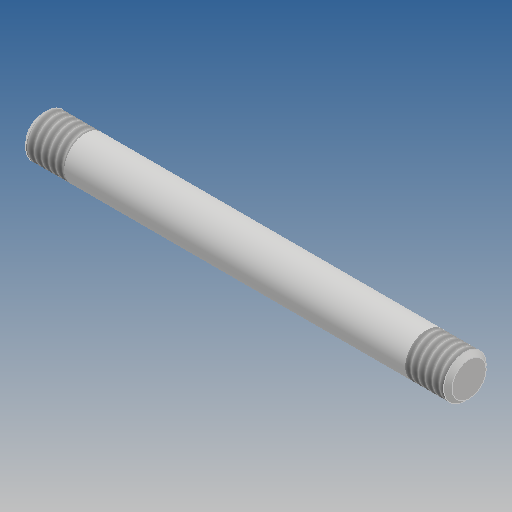
# Autodesk Inventor part: Pleuel
Saved by Autodesk Inventor 2018 (Build 220112000, 112)
## iProperties
Created: 2018-10-09
Part Number: Pleuel
Material: Generisch
Document SubType Name: Modeling
Designer: M.Knabel
Density: 1 g/cm^3
Appearance: Vorgabe
Mass: 0.211266 g
Surface Area: 2.93334 cm^2
Volume: 0.211266 cm^3
Author: M.Knabel
Autodesk Inventor part; units mm, degrees
ref_plane "YZ Plane" through (0, 0, 0) normal (1, 0, 0) x (0, 1, 0)
ref_plane "XZ Plane" through (0, 0, 0) normal (0, 1, 0) x (-1, 0, 0)
ref_plane "XY Plane" through (0, 0, 0) normal (0, 0, 1) x (1, 0, 0)
sketch "Skizze1" plane through (0, 0, 0) normal (0, 0, 1) x (1, 0, 0)
  line L0 (0, -0.3) -> (0, 1.8) projected
  line L1 (-6, 0) -> (36, 0) projected
  line L2 (0, 0) -> (30, 0)
  line L3 (30, 0) -> (30, 1.5)
  line L4 (30, 1.5) -> (0, 1.5)
  line L5 (0, 1.5) -> (0, 0)
  dimension "d0" = 3
  dimension "d1" = 30
  constraints: 8 end point, 2 parallel, 1 horizontal, 1 perpendicular
  measures "d0" diameter of L4 L1
  measures "d1" distance between parallel lines of L0 L3
revolve "Umdrehung1" add sketch "Skizze1" angle 360 about axis through (-10, 0, 0) along (1, 0, 0)
thread "Gewinde1" size "M3x0.5" class "6g" standard "ANSI Metric M Profile" length 3
thread "Gewinde2" size "M3x0.5" class "6g" standard "ANSI Metric M Profile" length 3
chamfer "Fase1" distance 0.3 angle 45 2 edges at (0, -1.5, 0) (30, -1.5, 0)
